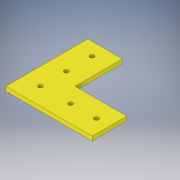
# Autodesk Inventor part: plate
Saved by Autodesk Inventor 2017 SP1 (Build 210196100, 196)
## iProperties
Created: 2018-01-30
Part Number: plate
Material: Aluminum 6061
Document SubType Name: Modeling
Designer: Ben
Density: 2.7 g/cm^3
Appearance: Canary
Author: Ben
Autodesk Inventor part; units mm, degrees
ref_plane "YZ Plane" through (0, 0, 0) normal (1, 0, 0) x (0, 1, 0)
ref_plane "XZ Plane" through (0, 0, 0) normal (0, 1, 0) x (-1, 0, 0)
ref_plane "XY Plane" through (0, 0, 0) normal (0, 0, 1) x (1, 0, 0)
sketch "Sketch1" plane through (0, 0, 0) normal (0, 1, 0) x (-1, 0, 0)
  circle A0 centre (0, 0) radius 1.5875
  line L0 (0, 0) -> (0, -38.1) construction
  circle A1 centre (-22.225, 0) radius 1.5875
  circle A2 centre (-41.275, 0) radius 1.5875
  circle A3 centre (0, -19.05) radius 1.5875
  circle A4 centre (0, -38.1) radius 1.5875
  line L1 (-12.7, -12.7) -> (-50.8, -12.7)
  line L2 (-50.8, -12.7) -> (-50.8, 12.7)
  line L3 (-50.8, 12.7) -> (12.7, 12.7)
  line L4 (12.7, 12.7) -> (12.7, -47.625)
  line L5 (12.7, -47.625) -> (-12.7, -47.625)
  line L6 (-12.7, -47.625) -> (-12.7, -12.7)
  line L7 (0, -38.1) -> (0, -47.625) construction
  line L8 (-41.275, 0) -> (-50.8, 0) construction
  line L9 (-12.7, -12.7) -> (-12.7, 12.7) construction
  line L10 (0, 0) -> (-41.275, 0) construction
  dimension "d0" = 3.175
  dimension "d1" = 22.225
  dimension "d2" = 25.4
  dimension "d3" = 9.525
  dimension "d4" = 19.05
  dimension "d5" = 19.05
  constraints: 22 end point, 8 perpendicular, 5 centre point, 4 equal radius, 3 midpoint, 2 coincident, 2 collinear, 2 horizontal, 2 point on line, 1 vertical
  measures "d0" diameter of A0
  measures "d1" distance of A1.centre point (0, 0)
  measures "d2" distance of L4.end L5.end
  measures "d3" distance of L7.start L7.end
  measures "d4" distance of L8.start A1.centre
  measures "d5" distance of L0.end A3.centre
extrude "Extrusion1" add sketch "Sketch1" along normal blind 3.175
body "Solid1"
